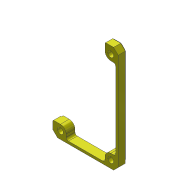
# Autodesk Inventor part: COXA_YAW_ROLL_ADPT_SPACER
Saved by Autodesk Inventor 2019.4 (Build 234330000, 330)
## iProperties
Created: 2019-11-06
Part Number: COXA_YAW_ROLL_ADPT_SPACER
Material: 一般
Document SubType Name: Modeling
Designer: y6tada
Density: 1 g/cm^3
Appearance: 滑らか - 黄
Author: y6tada
Autodesk Inventor part; units mm, degrees
ref_plane "YZ Plane" through (0, 0, 0) normal (1, 0, 0) x (0, 1, 0)
ref_plane "XZ Plane" through (0, 0, 0) normal (0, 1, 0) x (-1, 0, 0)
ref_plane "XY Plane" through (0, 0, 0) normal (0, 0, 1) x (1, 0, 0)
sketch "スケッチ1" plane through (0, 0, 0) normal (0, 0, 1) x (1, 0, 0)
  line L0 (8.75, 11.25) -> (12.25, 11.25)
  line L1 (14.25, 9.25) -> (14.25, -33.25)
  line L2 (12.25, -35.25) -> (-12.25, -35.25)
  line L3 (-14.25, -33.25) -> (-14.25, -29.75)
  line L4 (-12.25, 11.25) -> (-14.25, 9.25)
  line L5 (12.25, 11.25) -> (14.25, 9.25)
  line L6 (14.25, -33.25) -> (12.25, -35.25)
  line L7 (-12.25, -35.25) -> (-14.25, -33.25)
  line L8 (0, 0) -> (-26.5626, 0) construction
  line L9 (0, 0) -> (0, 27.9433) construction
  line L10 (-11, 8) -> (11, 8) construction
  line L11 (11, 8) -> (11, -32) construction
  line L12 (11, -32) -> (-11, -32) construction
  line L13 (-11, -32) -> (-11, 8) construction
  line L14 (-13.15, -28.5) -> (-13.15, 4.5) construction
  line L15 (-7.5, 10.15) -> (7.5, 10.15) construction
  line L16 (13.15, 4.5) -> (13.15, -28.5)
  line L17 (7.5, -34.15) -> (-7.5, -34.15)
  line L18 (8.5, 8) -> (8.5, 11)
  line L19 (11, 5.5) -> (12.15, 5.5)
  arc A0 (8.5, 8) -> (11, 5.5) centre (11, 8) ccw
  line L20 (12.15, -29.5) -> (11, -29.5)
  line L21 (8.5, -32) -> (8.5, -33.15)
  arc A1 (11, -29.5) -> (8.5, -32) centre (11, -32) ccw
  line L22 (-8.5, 8) -> (-8.5, 9.15) construction
  line L23 (-11, 5.5) -> (-12.15, 5.5) construction
  arc A2 (-11, 5.5) -> (-8.5, 8) centre (-11, 8) ccw construction
  line L24 (-14, -29.5) -> (-11, -29.5)
  line L25 (-8.5, -32) -> (-8.5, -33.15)
  arc A3 (-8.5, -32) -> (-11, -29.5) centre (-11, -32) ccw
  arc A4 (8.5, 9.15) -> (7.5, 10.15) centre (7.5, 9.15) ccw construction
  arc A5 (13.15, 4.5) -> (12.15, 5.5) centre (12.15, 4.5) ccw
  arc A6 (12.15, -29.5) -> (13.15, -28.5) centre (12.15, -28.5) ccw
  arc A7 (7.5, -34.15) -> (8.5, -33.15) centre (7.5, -33.15) ccw
  arc A8 (-8.5, -33.15) -> (-7.5, -34.15) centre (-7.5, -33.15) ccw
  arc A9 (-13.15, -28.5) -> (-12.15, -29.5) centre (-12.15, -28.5) ccw construction
  arc A10 (-12.15, 5.5) -> (-13.15, 4.5) centre (-12.15, 4.5) ccw construction
  arc A11 (-7.5, 10.15) -> (-8.5, 9.15) centre (-7.5, 9.15) ccw construction
  line L26 (8.75, 11.25) -> (8.5, 11)
  line L27 (-14, -29.5) -> (-14.25, -29.75)
  point P0 (-14.25, 11.25)
  point P1 (14.25, -35.25)
  point P2 (14.25, 11.25)
  point P3 (-14.25, -35.25)
  point P4 (8.5, 10.15)
  point P5 (13.15, 5.5)
  point P6 (13.15, -29.5)
  point P7 (8.5, -34.15)
  point P8 (-8.5, 10.15)
  point P9 (-13.15, 5.5)
  point P10 (-13.15, -29.5)
  point P11 (-8.5, -34.15)
  point P12 (8.5, 11.25)
  point P13 (-14.25, -29.5)
  dimension "d0" = 2
  dimension "d1" = 2
  dimension "d2" = 2
  dimension "d3" = 2
  dimension "d4" = 2
  dimension "d5" = 2
  dimension "d6" = 2
  dimension "d7" = 2
  dimension "d8" = 28.5
  dimension "d9" = 11.25
  dimension "d10" = 46.5
  dimension "d11" = 8
  dimension "d12" = 22
  dimension "d13" = 40
  dimension "d14" = 1.1
  dimension "d15" = 2.5
  dimension "d16" = 2.5
  dimension "d17" = 1.1
  dimension "d18" = 1.1
  dimension "d19" = 1
  dimension "d35" = 0.25
  dimension "d36" = 0.25
  dimension "d37" = 0.25
  dimension "d38" = 0.25
  constraints: 56 end point, 30 point on line, 24 point on circle, 20 tangent, 12 centre point, 10 symmetric about line, 7 coincident, 7 equal radius, 6 parallel, 6 perpendicular, 4 horizontal, 1 vertical, 5 other
  measures "d0" distance of L4.start point (-14.25, 11.25)
  measures "d1" distance of L4.end point (-14.25, 11.25)
  measures "d2" distance of L0.end point (14.25, 11.25)
  measures "d3" distance of L1.start point (14.25, 11.25)
  measures "d4" distance of L1.end point (14.25, -35.25)
  measures "d5" distance of L2.start point (14.25, -35.25)
  measures "d6" distance of L2.end point (-14.25, -35.25)
  measures "d7" distance of L3.start point (-14.25, -35.25)
  measures "d8" distance between parallel lines of L1 L3
  measures "d9" distance between parallel lines of L8 L0
  measures "d10" distance between parallel lines of L2 L0
  measures "d11" distance between parallel lines of L8 L10
  measures "d12" distance of L10.start L10.end
  measures "d13" distance of L12.end L10.start
  measures "d14" distance between parallel lines of L2 L17
  measures "d15" radius of A0
  measures "d16" radius of A1
  measures "d17" distance between parallel lines of L15 L0
  measures "d18" distance between parallel lines of L1 L16
  measures "d19" radius of A4
  measures "d35" distance of L0.start point (8.5, 11.25)
  measures "d36" distance of L18.end point (8.5, 11.25)
  measures "d37" distance of L24.start point (-14.25, -29.5)
  measures "d38" distance of L3.end point (-14.25, -29.5)
extrude "押し出し1" add sketch "スケッチ1" along normal blind 3.1
hole "穴1" at (-11, 8, 0) at (11, 8, 0) at (11, -32, 0) at (-11, -32, 0) direction (0, 0, 1) diameter 2.5 end through all
sketch "スケッチ3" plane through (0, 0, 0) normal (0, 0, -1) x (-1, 0, 0)
  line L0 (-8.75, 11.25) -> (-12.25, 11.25) construction
  line L1 (14.25, -33.25) -> (14.25, -29.75) construction
  line L2 (12.25, -35.25) -> (14.25, -33.25) construction
  line L3 (-12.25, -35.25) -> (12.25, -35.25) construction
  line L4 (-14.25, -33.25) -> (-12.25, -35.25) construction
  line L5 (-14.25, 9.25) -> (-14.25, -33.25) construction
  line L6 (-12.25, 11.25) -> (-14.25, 9.25) construction
  line L7 (-8.5, 10.625) -> (-11.087, 10.625)
  line L8 (-11.9911, 10.625) -> (-13.625, 8.9911) construction
  line L9 (-13.625, 8.087) -> (-13.625, -32.087)
  line L10 (-13.625, -32.9911) -> (-11.9911, -34.625) construction
  line L11 (-11.087, -34.625) -> (11.087, -34.625)
  line L12 (11.9911, -34.625) -> (13.625, -32.9911) construction
  line L13 (13.625, -32.087) -> (13.625, -29.5)
  line L14 (-13.1857, -33.1476) -> (-12.1476, -34.1857)
  line L15 (12.1476, -34.1857) -> (13.1857, -33.1476)
  line L16 (-13.1857, 9.1476) -> (-12.1476, 10.1857)
  arc A0 (-13.1857, 9.1476) -> (-13.625, 8.087) centre (-12.125, 8.087) ccw
  arc A1 (-11.087, 10.625) -> (-12.1476, 10.1857) centre (-11.087, 9.125) ccw
  arc A2 (13.1857, -33.1476) -> (13.625, -32.087) centre (12.125, -32.087) ccw
  arc A3 (11.087, -34.625) -> (12.1476, -34.1857) centre (11.087, -33.125) ccw
  arc A4 (-12.1476, -34.1857) -> (-11.087, -34.625) centre (-11.087, -33.125) ccw
  arc A5 (-13.625, -32.087) -> (-13.1857, -33.1476) centre (-12.125, -32.087) ccw
  arc A6 (-12.15, 5.5) -> (-13.15, 4.5) centre (-12.15, 4.5) ccw projected
  line L17 (-12.15, 5.5) -> (-11, 5.5) projected
  arc A7 (-11, 5.5) -> (-8.5, 8) centre (-11, 8) ccw projected
  line L18 (-8.5, 8) -> (-8.5, 11) construction
  line L19 (14, -29.5) -> (11, -29.5) construction
  arc A8 (11, -29.5) -> (8.5, -32) centre (11, -32) ccw projected
  line L20 (8.5, -32) -> (8.5, -33.15) projected
  arc A9 (7.5, -34.15) -> (8.5, -33.15) centre (7.5, -33.15) ccw projected
  circle A10 centre (11, -32) radius 1.25 projected
  line L21 (7.5, -34.15) -> (-7.5, -34.15) projected
  arc A11 (-8.5, -33.15) -> (-7.5, -34.15) centre (-7.5, -33.15) ccw projected
  line L22 (-8.5, -33.15) -> (-8.5, -32) projected
  arc A12 (-8.5, -32) -> (-11, -29.5) centre (-11, -32) ccw projected
  line L23 (-11, -29.5) -> (-12.15, -29.5) projected
  arc A13 (-13.15, -28.5) -> (-12.15, -29.5) centre (-12.15, -28.5) ccw projected
  circle A14 centre (-11, -32) radius 1.25 projected
  line L24 (-13.15, -28.5) -> (-13.15, 4.5) projected
  circle A15 centre (-11, 8) radius 1.25 projected
  line L25 (11, -29.5) -> (13.625, -29.5)
  line L26 (-8.5, 8) -> (-8.5, 10.625)
  point P0 (0, 0)
  dimension "d30" = 0.625
  dimension "d31" = 1.5
  dimension "d32" = 0.2
  dimension "d39" = 0.625
  dimension "d40" = 0.625
  dimension "d41" = 0.2
  constraints: 24 end point, 12 point on circle, 12 tangent, 8 point on line, 6 centre point, 4 equal radius, 3 parallel, 2 perpendicular, 1 collinear, 1 vertical, 4 other
  measures "d30" distance between parallel lines of L0 L7
  measures "d31" radius of A0
  measures "d32" distance between parallel lines of L14 L10
  measures "d39" distance between parallel lines of L4 L10
  measures "d40" distance between parallel lines of L1 L13
  measures "d41" distance between parallel lines of L12 L15
extrude "押し出し2" add sketch "スケッチ3" along normal blind 0.75
equation "\"d1\" = d0"
equation "\"d2\" = d0"
equation "\"d3\" = d2"
equation "\"d4\" = d0"
equation "\"d5\" = d4"
equation "\"d6\" = d0"
equation "\"d7\" = d6"
equation "\"d36\" = d35"
equation "\"d37\" = d35"
equation "\"d38\" = d37"
